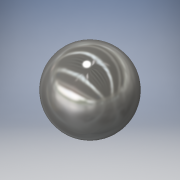
# Autodesk Inventor part: NATHAN BALL
Saved by Autodesk Inventor 2016 (Build 200138000, 138)
## iProperties
Created: 2016-10-13
Part Number: NATHAN BALL
Material: Generic
Document SubType Name: Modeling
Designer: brandn
Density: 1 g/cm^3
Appearance: Default
Author: brandn
Autodesk Inventor part; units mm, degrees
ref_plane "YZ Plane" through (0, 0, 0) normal (1, 0, 0) x (0, 1, 0)
ref_plane "XZ Plane" through (0, 0, 0) normal (0, 1, 0) x (-1, 0, 0)
ref_plane "XY Plane" through (0, 0, 0) normal (0, 0, 1) x (1, 0, 0)
sketch "Sketch1" plane through (0, 0, 0) normal (1, 0, 0) x (0, 1, 0)
  arc A0 (8.7249, 0) -> (-8.7249, 0) centre (0, 0) ccw
  line L0 (8.7249, 0) -> (-8.7249, 0)
  dimension "d0" = 17.4498
  constraints: 2 end point, 2 point on circle, 1 centre point, 1 coincident, 1 horizontal
  measures "d0" diameter of A0
revolve "Revolution1" add sketch "Sketch1" angle 360 about axis through (0, 8.7249, 0) along (0, -1, 0)
body "Solid1"
